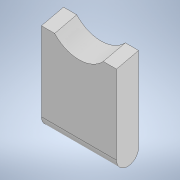
# Autodesk Inventor part: Block
Saved by Autodesk Inventor 2021 (Build 250183000, 183)
## iProperties
Created: 2021-04-12
Part Number: Block
Material: Generic
Document SubType Name: Modeling
Designer: Nabeel Azafer
Density: 1 g/cm^3
Appearance: Default
Author: Nabeel Azafer
Autodesk Inventor part; units mm, degrees
ref_plane "YZ Plane" through (0, 0, 0) normal (1, 0, 0) x (0, 1, 0)
ref_plane "XZ Plane" through (0, 0, 0) normal (0, 1, 0) x (-1, 0, 0)
ref_plane "XY Plane" through (0, 0, 0) normal (0, 0, 1) x (1, 0, 0)
sketch "Sketch1" plane through (0, 0, 0) normal (0, 0, 1) x (1, 0, 0)
  line L0 (0, 0) -> (17, 0)
  line L1 (17, 0) -> (17, 21.5)
  line L2 (17, 21.5) -> (0, 21.5)
  line L3 (0, 21.5) -> (0, 0)
  dimension "d0" = 17
  dimension "d1" = 21.5
  constraints: 8 end point, 2 parallel, 1 horizontal, 1 perpendicular
  measures "d0" distance of L0.start L0.end
  measures "d1" distance of L2.end L0.start
extrude "Extrusion1" add sketch "Sketch1" along normal blind 5
fillet "Fillet2" radius 2.5 2 edges at (8.5, 0, 5) (8.5, 0, 0)
ref_plane "Work Plane1" through (8.5, 21.5, 0) normal (-1, 0, 0) x (0, 0, 1)
sketch "Sketch5" plane through (8.5, 21.5, 0) normal (-1, 0, 0) x (0, 0, 1)
  line L0 (0, 0) -> (5, -1.1543)
  line L1 (5, -19) -> (5, 0) projected
  line L2 (0, 0) -> (5.1315, 0) construction
  point P0 (0, -21.5)
  dimension "d22" = 13
  constraints: 4 end point, 1 equal length, 1 horizontal, 1 point on line
  measures "d22" angle of L0 L2
sketch "Sketch6" plane through (0, 0, 0) normal (0, 0, -1) x (-1, 0, 0)
  line L0 (-14, 21.5) -> (-14, 24.5)
  line L1 (-14, 24.5) -> (-3, 24.5)
  line L2 (-3, 24.5) -> (-3, 21.5)
  line L3 (-17, 21.5) -> (0, 21.5) projected
  arc A0 (-14, 21.5) -> (-3, 21.5) centre (-8.5, 26.599) ccw
  point P0 (0, 0)
  dimension "d27" = 3
  dimension "d31" = 3
  dimension "d32" = 3
  dimension "d33" = 3
  dimension "d34" = 7.5
  constraints: 6 end point, 2 perpendicular, 2 point on circle, 1 centre point, 1 vertical
  measures "d27" distance of L0.start L0.end
  measures "d31" distance from line of L3.end L2
  measures "d32" distance between parallel lines of L3 L1
  measures "d33" distance of L1.end L2.end
  measures "d34" radius of A0
sweep "Sweep1" cut profiles "Sketch6" path "Sketch5" path curves L0
sketch "Sketch8" plane through (17, 21.5, 5) normal (1, 0, 0) x (0, 0, -1)
  line L0 (5, 0) -> (0, 0) projected
  line L1 (5, 0) -> (0, -1.1543) projected
  line L2 (5, 0) -> (0, -1.1543)
  line L3 (0, -19) -> (0, 0) projected
  line L4 (0, -1.1543) -> (0, 0)
  line L5 (0, 0) -> (5, 0)
  point P0 (5, -21.5)
  constraints: 6 end point, 2 collinear, 1 perpendicular
extrude "Extrusion6" cut sketch "Sketch8" against normal blind 17
body "Solid1"
